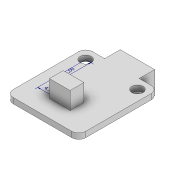
# Autodesk Inventor part: Temp_Module
Saved by Autodesk Inventor 2021.2 (Build 252289000, 289)
## iProperties
Created: 2023-12-05
Part Number: Temp_Module
Material: Типовые
Document SubType Name: Modeling
Designer: Egor
Density: 1 g/cm^3
Appearance: По умолчанию
Author: Egor
Autodesk Inventor part; units mm, degrees
ref_plane "YZ Plane" through (0, 0, 0) normal (1, 0, 0) x (0, 1, 0)
ref_plane "XZ Plane" through (0, 0, 0) normal (0, 1, 0) x (-1, 0, 0)
ref_plane "XY Plane" through (0, 0, 0) normal (0, 0, 1) x (1, 0, 0)
sketch "Эскиз1" plane through (0, 0, 0) normal (0, 1, 0) x (-1, 0, 0)
  line L0 (2, 0) -> (19, 0)
  line L1 (21, -2) -> (21, -21)
  line L2 (19, -23) -> (2, -23)
  line L3 (0, -21) -> (0, -2)
  circle A0 centre (18, -20) radius 1.6
  circle A1 centre (3, -20) radius 1.6
  arc A2 (19, -23) -> (21, -21) centre (19, -21) ccw
  arc A3 (0, -21) -> (2, -23) centre (2, -21) ccw
  arc A4 (2, 0) -> (0, -2) centre (2, -2) ccw
  arc A5 (21, -2) -> (19, 0) centre (19, -2) ccw
  point P0 (0, 0)
  dimension "d6" = 2
  dimension "d20" = 15
  dimension "d21" = 3
  dimension "d22" = 3
  constraints: 8 end point, 8 point on circle, 8 tangent, 6 centre point, 3 equal radius, 2 parallel, 2 point on line, 1 horizontal, 1 perpendicular
  measures "d6" radius of A2
  measures "d20" distance of A0.centre A1.centre
  measures "d21" distance from line of L2 A1.centre
  measures "d22" distance from line of L3 A1.centre
extrude "Выдавливание1" add sketch "Эскиз1" along normal blind 1.6
sketch "Эскиз2" plane through (0, 1.6, 0) normal (0, 1, 0) x (1, 0, 0)
  circle A0 centre (-18, 20) radius 1.6 projected
  circle A1 centre (-3, 20) radius 1.6 projected
  line L0 (-10.5, 27.5) -> (-5.5, 27.5)
  line L1 (-5.5, 27.5) -> (-15.5, 27.5)
  line L2 (-15.5, 27.5) -> (-5.5, 27.5)
  line L3 (-5.5, 27.5) -> (-5.5, 20)
  line L4 (-5.5, 20) -> (-15.5, 20)
  line L5 (-15.5, 20) -> (-15.5, 27.5)
  point P0 (0, 0)
  constraints: 12 end point, 2 parallel, 1 horizontal, 1 perpendicular, 1 point on line
extrude "Выдавливание2" add sketch "Эскиз2" against normal blind 6.5 contours L0 L3 L4 L5 L1
sketch "Эскиз3" plane through (0, 1.6, 0) normal (0, 1, 0) x (1, 0, 0)
  line L0 (-5.5, 20) -> (-15.5, 20) projected
  line L1 (-10.5, 20) -> (-10.5, 5)
  line L2 (-10.5, 5) -> (-13.5, 5)
  line L3 (-10.5, 5) -> (-7.5, 5)
  line L4 (-13.5, 5) -> (-7.5, 5)
  line L5 (-7.5, 5) -> (-7.5, 9)
  line L6 (-7.5, 9) -> (-13.5, 9)
  line L7 (-13.5, 9) -> (-13.5, 5)
  line L8 (-21, 21) -> (-21, 2) projected
  line L9 (0, 2) -> (0, 21) projected
  point P0 (0, 0)
  dimension "d14" = 15
  dimension "d15" = 3
  dimension "d16" = 3
  dimension "d17" = 4
  dimension "d23" = 7.5
  dimension "d24" = 7.5
  constraints: 14 end point, 2 horizontal, 2 parallel, 2 perpendicular, 1 midpoint, 1 vertical
  measures "d14" distance of L1.start L1.end
  measures "d15" distance of L1.end L2.end
  measures "d16" distance of L1.end L3.end
  measures "d17" distance of L5.end L4.end
  measures "d23" distance between parallel lines of L8 L7
  measures "d24" distance between parallel lines of L9 L5
extrude "Выдавливание3" add sketch "Эскиз3" along normal blind 5
